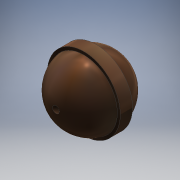
# Autodesk Inventor part: caramelo
Saved by Autodesk Inventor 2016 (Build 200138000, 138)
## iProperties
Created: 2016-02-19
Part Number: caramelo
Material: Genérico
Document SubType Name: Modeling
Designer: Usuario1
Density: 1 g/cm^3
Appearance: Valor por defecto
Author: Usuario1
Autodesk Inventor part; units mm, degrees
ref_plane "YZ Plane" through (0, 0, 0) normal (1, 0, 0) x (0, 1, 0)
ref_plane "XZ Plane" through (0, 0, 0) normal (0, 1, 0) x (-1, 0, 0)
ref_plane "XY Plane" through (0, 0, 0) normal (0, 0, 1) x (1, 0, 0)
sketch "Boceto1" plane through (0, 0, 0) normal (0, 0, 1) x (1, 0, 0)
  line L0 (-5.35, -5) -> (-5.35, -5.9)
  line L1 (-5.35, -5.9) -> (-4.9183, -5.9)
  line L2 (-5.35, -5) -> (-5.35, -4.1)
  line L3 (-5.35, -4.1) -> (-4.9183, -4.1)
  line L4 (-0.5, -4.9) -> (-0.5, -9.9749)
  line L5 (0, -4.9) -> (-0.5, -4.9)
  arc A0 (0, 0) -> (-4.9183, -4.1) centre (0, -5) ccw
  arc A1 (-4.9183, -5.9) -> (-0.5, -9.9749) centre (0, -5) ccw
  line L6 (0, -4.9) -> (0, 0)
  point P0 (0, 0)
  constraints: 14 end point, 4 point on circle, 2 centre point
revolve "Revolución1" add sketch "Boceto1" angle 360 about axis through (0, -4.9, 0) along (0, 1, 0)
